# Autodesk Inventor part: Center Rod
Saved by Autodesk Inventor 2014 SP1 (Build 180222100, 222)
## iProperties
Created: 2014-04-09
Part Number: Center Rod
Material: Generic
Document SubType Name: Modeling
Designer: tom
Density: 1 g/cm^3
Appearance: Default
Author: tom
Autodesk Inventor part; units mm, degrees
ref_plane "YZ Plane" through (0, 0, 0) normal (1, 0, 0) x (0, 1, 0)
ref_plane "XZ Plane" through (0, 0, 0) normal (0, 1, 0) x (-1, 0, 0)
ref_plane "XY Plane" through (0, 0, 0) normal (0, 0, 1) x (1, 0, 0)
ref_plane "Work Plane1" through (73.7063, 178.9516, -43.9883) normal (0, 0, 1) x (1, 0, 0)
sketch "Sketch1" plane through (73.7063, 178.9516, -43.9883) normal (0, 0, 1) x (1, 0, 0)
  circle A0 centre (-63.5, 63.5) radius 3.175 projected
ref_plane "Work Plane2" through (15.6318, 236.9932, 289.0057) normal (0, 0, 1) x (1, 0, 0)
sketch "Sketch2" plane through (15.6318, 236.9932, 289.0057) normal (0, 0, 1) x (1, 0, 0)
  circle A0 centre (0.9245, -0.8916) radius 3.175 projected
loft "Loft1" add profiles "Sketch1", "Sketch2"
body "Solid1"
